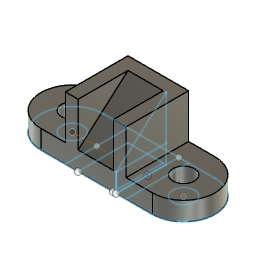
A2 (Autodesk Fusion 360 design; units mm, degrees)
Autodesk Fusion 360 part; units mm, degrees
sketch "BaseSketch" plane through (0, 0, 0) normal (0, 0, 1) x (1, 0, 0)
  line L0 (-77, -32) -> (37, -32)
  arc A0 (37, -32) -> (37, 32) centre (37, 0) ccw
  line L1 (37, 32) -> (-77, 32)
  arc A1 (-77, 32) -> (-77, -32) centre (-77, 0) ccw
  line L2 (-77, 0) -> (37, 0) construction
  circle A2 centre (-77, 0) radius 11
  circle A3 centre (37, 0) radius 11
  line L3 (-77, 0) -> (-52, 0) construction
  line L4 (-52, 32) -> (10, 32) construction
  line L5 (10, 32) -> (10, -32)
  line L6 (10, -32) -> (-52, -32) construction
  line L7 (-52, -32) -> (-52, 32)
  line L8 (-39, -32) -> (-39, 19)
  line L9 (-39, 19) -> (-3, 19)
  line L10 (-3, 19) -> (-3, -32)
  dimension "d2" = 64
  dimension "d3" = 22
  dimension "d4" = 22
  dimension "d5" = 25
  dimension "d6" = 62
  dimension "d7" = 13
  constraint tangent L0 A0
  constraint tangent A0 L1
  constraint parallel L0 L1
  constraint tangent L1 A1
  constraint tangent L0 A1
  constraint concentric A1 A2
  constraint concentric A0 A3
  constraint coincident A1.centre L2.start
  constraint parallel L2 L3
  constraint horizontal L4
  constraint vertical L5
  constraint horizontal L6
  constraint vertical L7
  constraint coincident L0 L5.end
  constraint coincident L1 L4.start
  measures "d2" diameter of A0
  measures "d3" diameter of A2
  measures "d4" diameter of A3
  measures "d5" distance of A1.centre L3.end
  measures "d6" distance of L4.start L4.end
extrude "Extrude1" add sketch "BaseSketch" along normal blind 19 contours L0 L1 A1 L7 | L0 A0 L1 L5 makes body 1 at (15.3333, 0, 0) makes body 2 at (-66.8333, 24.5088, 0)
extrude "Extrude2" add sketch "BaseSketch" along normal blind 64 contours L0 L1 L5 L7 L8 L9 L10 bodies 1 2
extrude "Extrude3" add sketch "BaseSketch" along normal blind 19 contours L0 L8 L9 L10 bodies 1
sketch "TriangleSketch" plane through (0, 0, 0) normal (1, 0, 0) x (0, 1, 0)
  line L0 (32, 0) -> (19, 0)
  line L1 (19, 0) -> (-32, 0)
  line L2 (19, 0) -> (-32, 0)
  line L3 (-32, 0) -> (-32, 19)
  line L4 (-32, 19) -> (19, 19)
  line L5 (19, 19) -> (19, 0)
  line L6 (19, 19) -> (19, 64)
  line L7 (19, 64) -> (-32, 19)
  dimension "d14" = 13
  dimension "d15" = 51
  dimension "d16" = 19
  constraint horizontal L0
  constraint parallel L0 L1
  constraint horizontal L2
  constraint vertical L3
  constraint horizontal L4
  constraint vertical L5
  constraint perpendicular L4 L6
  measures "d14" distance of L0.start L0.end
  measures "d15" distance of L0.end L1.end
  measures "d16" distance of L0.end L4.end
extrude "Extrude4" add sketch "TriangleSketch" against normal blind 36 from surface at -3 contours L4 L6 L7 bodies 1
named bodies: "MainBodyA2"
